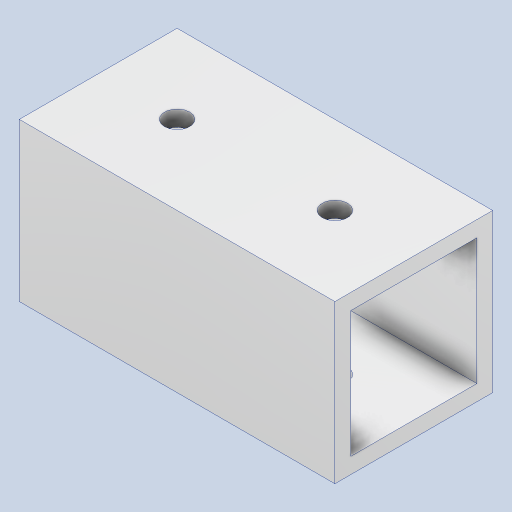
# Autodesk Inventor part: arm_jig
Saved by Autodesk Inventor 2024 (Build 280153000, 153)
## iProperties
Company: 細田研究室
Created: 2025-06-20
Part Number: arm_jig
Material: アルミニウム 6061
Document SubType Name: Modeling
Designer: Mizuki Yoshida
Density: 2.7 g/cm^3
Appearance: アルミニウム - フラット
個数: 4
Author: Mizuki Yoshida
Autodesk Inventor part; units mm, degrees
ref_plane "YZ Plane" through (0, 0, 0) normal (1, 0, 0) x (0, 1, 0)
ref_plane "XZ Plane" through (0, 0, 0) normal (0, 1, 0) x (-1, 0, 0)
ref_plane "XY Plane" through (0, 0, 0) normal (0, 0, 1) x (1, 0, 0)
sketch "スケッチ1" plane through (0, 0, 0) normal (0, 1, 0) x (-1, 0, 0)
  line L0 (0, 0) -> (-20, 0)
  line L1 (-20, 0) -> (-20, -20)
  line L2 (-20, -20) -> (0, -20)
  line L3 (0, -20) -> (0, 0)
  line L4 (-2, -2) -> (-18, -2)
  line L5 (-18, -2) -> (-18, -18)
  line L6 (-18, -18) -> (-2, -18)
  line L7 (-2, -18) -> (-2, -2)
  dimension "d0" = 20
  dimension "d1" = 20
  dimension "d2" = 16
  dimension "d3" = 16
  dimension "d4" = 2
  dimension "d18" = 2
  constraints: 16 end point, 4 parallel, 2 horizontal, 2 perpendicular
  measures "d0" distance of L2.end L1.end
  measures "d1" distance of L1.end L0.end
  measures "d2" distance of L4.end L5.end
  measures "d3" distance of L5.end L6.end
  measures "d4" distance between parallel lines of L2 L6
  measures "d18" distance between parallel lines of L3 L7
extrude "押し出し1" add sketch "スケッチ1" along normal blind 40
sketch "スケッチ2" plane through (0, 0, 0) normal (0, 0, 1) x (1, 0, 0)
  line L0 (20, 0) -> (20, 40) projected
  line L1 (0, 0) -> (20, 0) projected
  line L2 (0, 40) -> (20, 40) projected
  point P0 (10, 30)
  point P1 (10, 10)
  dimension "d7" = 10
  dimension "d8" = 10
  dimension "d9" = 10
  dimension "d10" = 10
  measures "d7" distance from line of L0 point (10, 30)
  measures "d8" distance from line of L0 point (10, 10)
  measures "d9" distance from line of L1 point (10, 10)
  measures "d10" distance from line of point (10, 30) L2
hole "穴1" at (10, 30, 0) at (10, 10, 0) direction (0, 0, -1) diameter 3.2 end through all
